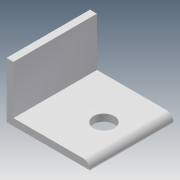
# Autodesk Inventor part: axlesupport end
Saved by Autodesk Inventor 2014 (Build 180170000, 170)
## iProperties
Created: 2016-01-12
Part Number: axlesupport end
Material: Steel, Mild
Document SubType Name: Modeling
Designer: Paul
Density: 7.86 g/cm^3
Appearance: Steel
Mass: 66.3586 g
Surface Area: 61.1015 cm^2
Volume: 8.44257 cm^3
Author: Paul
Autodesk Inventor part; units mm, degrees
ref_plane "YZ Plane" through (0, 0, 0) normal (1, 0, 0) x (0, 1, 0)
ref_plane "XZ Plane" through (0, 0, 0) normal (0, 1, 0) x (-1, 0, 0)
ref_plane "XY Plane" through (0, 0, 0) normal (0, 0, 1) x (1, 0, 0)
sketch "Sketch1" plane through (0, 0, 0) normal (0, 0, 1) x (1, 0, 0)
  line L0 (0, 0) -> (0, 38.1)
  line L1 (0, 0) -> (38.1, 0)
  line L2 (34.925, 3.175) -> (3.175, 3.175)
  line L3 (3.175, 3.175) -> (3.175, 34.925)
  arc A0 (3.175, 34.925) -> (0, 38.1) centre (0, 34.925) ccw
  arc A1 (38.1, 0) -> (34.925, 3.175) centre (34.925, 0) ccw
  dimension "d0" = 38.1
  dimension "d1" = 38.1
  dimension "d2" = 3.175
  constraints: 8 end point, 6 point on circle, 4 point on line, 2 centre point, 2 perpendicular, 1 vertical
  measures "d0" distance of L0.start L0.end
  measures "d1" distance of L0.start L1.end
  measures "d2" distance between parallel lines of L2 L1
extrude "Extrusion1" add sketch "Sketch1" along normal blind 38.1
sketch "Sketch2" plane through (0, 0, 0) normal (0, -1, 0) x (1, 0, 0)
  line L0 (38.1, 0) -> (38.1, 38.1) projected
  circle A0 centre (25.4, 19.05) radius 4.7625
  dimension "d5" = 9.525
  dimension "d6" = 12.7
  constraints: 1 centre point
  measures "d5" diameter of A0
  measures "d6" distance from line of A0.centre L0
extrude "Extrusion2" cut sketch "Sketch2" against normal blind 38.1
sketch "Sketch3" plane through (0, 0, 0) normal (-1, 0, 0) x (0, 0, 1)
  line L0 (0, 38.1) -> (0, 0) projected
  line L1 (38.1, 38.1) -> (38.1, 0) projected
  line L2 (0, 38.1) -> (38.1, 38.1) projected
  line L3 (0, 25.4) -> (38.1, 25.4)
  dimension "d9" = 12.7
  constraints: 2 end point, 2 point on line, 1 parallel
  measures "d9" distance between parallel lines of L3 L2
extrude "Extrusion3" cut sketch "Sketch3" against normal blind 38.1
body "Solid1"
